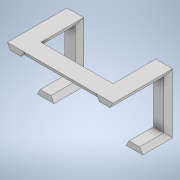
# Autodesk Inventor part: HexWeaponGuard
Saved by Autodesk Inventor 2020 (Build 240168000, 168)
## iProperties
Created: 2024-01-16
Part Number: HexWeaponGuard
Material: Generic
Document SubType Name: Modeling
Designer: smz3rm
Density: 1 g/cm^3
Appearance: Default
Author: smz3rm
Autodesk Inventor part; units mm, degrees
ref_plane "YZ Plane" through (0, 0, 0) normal (1, 0, 0) x (0, 1, 0)
ref_plane "XZ Plane" through (0, 0, 0) normal (0, 1, 0) x (-1, 0, 0)
ref_plane "XY Plane" through (0, 0, 0) normal (0, 0, 1) x (1, 0, 0)
sketch "Sketch1" plane through (0, 0, 0) normal (0, 1, 0) x (-1, 0, 0)
  line L0 (59, 4.4952) -> (-59, 4.4952)
  line L1 (-59, 4.4952) -> (-59, -4.4952)
  line L2 (-59, -4.4952) -> (59, -4.4952)
  line L3 (59, -4.4952) -> (59, 4.4952)
  line L4 (59, 4.4952) -> (-59, -4.4952) construction
  line L5 (-59, 4.4952) -> (59, -4.4952) construction
  line L6 (43.4282, -4.4952) -> (38.2376, 4.4952)
  line L7 (38.2376, 4.4952) -> (43.4282, 13.4856)
  line L8 (43.4282, 13.4856) -> (53.8094, 13.4856)
  line L9 (53.8094, 13.4856) -> (59, 4.4952)
  line L10 (59, 4.4952) -> (53.8094, -4.4952)
  line L11 (53.8094, -4.4952) -> (43.4282, -4.4952)
  line L12 (26.5875, 4.4952) -> (21.3969, -4.4952)
  line L13 (11.0157, -4.4952) -> (5.8251, 4.4952)
  line L14 (21.3969, -4.4952) -> (11.0157, -4.4952)
  line L15 (-5.8251, 4.4952) -> (-11.0157, -4.4952)
  line L16 (-21.3969, -4.4952) -> (-26.5875, 4.4952)
  line L17 (-11.0157, -4.4952) -> (-21.3969, -4.4952)
  line L18 (-38.2376, 4.4952) -> (-43.4282, -4.4952)
  line L19 (-53.8094, -4.4952) -> (-59, 4.4952)
  line L20 (-43.4282, -4.4952) -> (-53.8094, -4.4952)
  line L21 (59, 4.4952) -> (-59, 4.4952)
  line L22 (-59, 4.4952) -> (-59, 8.4952)
  line L23 (-59, 8.4952) -> (59, 8.4952)
  line L24 (59, 8.4952) -> (59, 4.4952)
  line L25 (41.4282, -4.4952) -> (36.2376, 4.4952)
  line L26 (28.5875, 4.4952) -> (23.3969, -4.4952)
  line L27 (38.547, 0.4952) -> (26.2781, 0.4952)
  line L28 (0, -8.0913) -> (0, 17.0817) projected
  line L29 (-41.4282, -4.4952) -> (-36.2376, 4.4952)
  line L30 (-28.5875, 4.4952) -> (-23.3969, -4.4952)
  line L31 (-38.547, 0.4952) -> (-26.2781, 0.4952)
  point P0 (0, 0)
  point P1 (48.6188, 4.4952)
  point P2 (-36.2376, 4.4952)
  point P3 (36.2376, 4.4952)
  dimension "d0" = 118
  dimension "d1" = 8.9904
  dimension "d4" = 32.4125
  dimension "d9" = 4
  dimension "d10" = 2
  dimension "d11" = 2
  dimension "d12" = 4
  constraints: 62 end point, 11 point on line, 6 parallel, 6 symmetric about line, 4 horizontal, 2 midpoint, 2 perpendicular, 1 collinear, 34 other
  measures "d0" distance of L2.end L1.end
  measures "d1" distance between parallel lines of L0 L2
  measures "d4" distance of L0.start L12.start
  measures "d9" distance of L21.end L22.end
  measures "d10" distance of L6.start L25.start
  measures "d11" distance of L12.end L26.end
  measures "d12" distance between parallel lines of L0 L27
extrude "Extrusion1" add sketch "Sketch1" along normal blind 43.6188 contours L25 L27 L26 L0 | L0 L30 L31 L29
sketch "Sketch2" plane through (-26.2781, 0, 0.4952) normal (0, 0, -1) x (-1, 0, 0)
  line L0 (9.9595, 43.6188) -> (2.3094, 43.6188) projected
  line L1 (2.3094, 39.6188) -> (9.9595, 39.6188)
  line L2 (9.9595, 39.6188) -> (12.2689, 43.6188)
  line L3 (2.3094, 39.6188) -> (0, 43.6188)
  line L4 (0, 43.6188) -> (12.2689, 43.6188) projected
  line L5 (-26.2781, -8.7238) -> (-26.2781, 52.3426) projected
  line L6 (-54.8655, 39.6188) -> (-62.5157, 39.6188)
  line L7 (-62.5157, 39.6188) -> (-64.8251, 43.6188)
  line L8 (-54.8655, 39.6188) -> (-52.5561, 43.6188)
  line L9 (-64.8251, 43.6188) -> (-52.5561, 43.6188) projected
  line L10 (-64.8251, 0) -> (-64.8251, 43.6188) projected
  line L11 (-64.8251, 21.8094) -> (12.2689, 21.8094)
  line L12 (12.2689, 0) -> (12.2689, 43.6188) projected
  line L13 (9.9595, 0) -> (2.3094, 0)
  line L14 (2.3094, 4) -> (9.9595, 4)
  line L15 (9.9595, 4) -> (12.2689, 0)
  line L16 (2.3094, 4) -> (0, 0)
  line L17 (0, 0) -> (12.2689, 0)
  line L18 (-54.8655, 4) -> (-52.5561, 0)
  line L19 (-54.8655, 4) -> (-62.5157, 4)
  line L20 (-62.5157, 4) -> (-64.8251, 0)
  line L21 (-64.8251, 0) -> (-52.5561, 0)
  point P0 (-26.2781, 0)
  dimension "d15" = 4
  dimension "d18" = 7.6501
  dimension "d20" = 12.2689
  constraints: 32 end point, 12 symmetric about line, 2 midpoint, 2 vertical alignment, 1 horizontal
  measures "d15" distance between parallel lines of L4 L1
  measures "d18" distance of L1.start L1.end
  measures "d20" distance of L7.end L8.end
extrude "Extrusion2" add sketch "Sketch2" against normal blind 43.5048
sketch "Sketch3" plane through (0, 0, 0) normal (1, 0, 0) x (0, 1, 0)
  line L0 (43.6188, 44) -> (39.6188, 41.6906)
  line L1 (39.6188, 34.0405) -> (43.6188, 31.7311)
  line L2 (43.6188, 0.4952) -> (43.6188, 44) projected
  line L3 (39.6188, 4.4952) -> (39.6188, 44) projected
  line L4 (43.6188, 31.7311) -> (43.6188, 44)
  line L5 (39.6188, 34.0405) -> (39.6188, 41.6906)
  line L6 (39.6188, 37.8655) -> (43.6188, 37.8655)
  point P0 (0, 0)
  dimension "d21" = 12.2689
  dimension "d22" = 7.6501
  constraints: 10 end point, 2 midpoint, 2 point on line, 1 collinear, 1 parallel, 1 perpendicular
  measures "d21" distance of L0.start L1.end
  measures "d22" distance of L0.end L1.start
extrude "Extrusion3" add sketch "Sketch3" along normal through all both and the other way through all
sketch "Sketch6" plane through (-26.2781, 0, 44) normal (0, 0, 1) x (1, 0, 0)
  line L0 (-9.9595, 4) -> (-12.2689, 0) projected
  line L1 (-12.2689, 0) -> (0, 0) projected
  line L2 (0, 0) -> (-2.3094, 4) projected
  line L3 (-2.3094, 4) -> (-9.9595, 4) projected
  line L4 (52.5561, 0) -> (64.8251, 0) projected
  line L5 (64.8251, 0) -> (62.5157, 4) projected
  line L6 (62.5157, 4) -> (54.8655, 4) projected
  line L7 (54.8655, 4) -> (52.5561, 0) projected
  point P0 (26.2781, 0)
extrude "Extrusion4" cut sketch "Sketch6" against normal blind 21.7524
equation "\"d0\" = BodyWidth"
equation "\"d1\" = RidgeHeight"
equation "\"d4\" = RidgeSpacing"
equation "\"d9\" = SideThickness"
equation "\"d12\" = SideThickness"
equation "\"d15\" = SideThickness"
equation "\"d16\" = 0.5 * FlipperArmLength"
equation "\"d21\" = d20"
equation "\"d22\" = d18"
equation "\"d25\" = 0.25 * FlipperArmLength"
equation "\"RidgeHeight\" = 0.433013 * RidgeLength"
equation "\"BodyWidth\" = 118"
equation "\"RidgeSpacing\" = 32.412535"
equation "\"SideThickness\" = 4"
equation "\"FlipperArmLength\" = 87.009619"
equation "\"RidgeLength\" = 20.762396"
body "Solid1"
